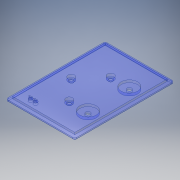
# Autodesk Inventor part: top
Saved by Autodesk Inventor 2017 SP1 (Build 210196100, 196)
## iProperties
Created: 2016-12-24
Part Number: top
Material: Generic
Document SubType Name: Modeling
Designer: wsh32
Density: 1 g/cm^3
Appearance: Clear - Blue
Author: wsh32
Autodesk Inventor part; units mm, degrees
ref_plane "YZ Plane" through (0, 0, 0) normal (1, 0, 0) x (0, 1, 0)
ref_plane "XZ Plane" through (0, 0, 0) normal (0, 1, 0) x (-1, 0, 0)
ref_plane "XY Plane" through (0, 0, 0) normal (0, 0, 1) x (1, 0, 0)
sketch "Sketch1" plane through (0, 0, 0) normal (0, 1, 0) x (-1, 0, 0)
  line L0 (0, 0) -> (-106.68, 0)
  line L1 (-106.68, 0) -> (-106.68, -153.67)
  line L2 (-106.68, -153.67) -> (0, -153.67)
  line L3 (0, -153.67) -> (0, 0)
  dimension "d0" = 153.67
  dimension "d1" = 106.68
  constraints: 8 end point, 2 parallel, 1 horizontal, 1 perpendicular
  measures "d0" distance of L2.end L0.start
  measures "d1" distance of L1.end L2.end
extrude "Extrusion1" add sketch "Sketch1" along normal blind 3.175
sketch "Sketch2" plane through (0, 3.175, 0) normal (0, 1, 0) x (1, 0, 0)
  line L0 (0, 0) -> (106.68, 0) projected
  line L1 (106.68, 0) -> (106.68, 153.67) projected
  line L2 (106.68, 153.67) -> (0, 153.67) projected
  line L3 (0, 153.67) -> (0, 0) projected
  line L4 (5.08, 5.08) -> (101.6, 5.08)
  line L5 (101.6, 5.08) -> (101.6, 148.59)
  line L6 (101.6, 148.59) -> (5.08, 148.59)
  line L7 (5.08, 148.59) -> (5.08, 5.08)
  dimension "d4" = 5.08
  constraints: 8 end point, 3 other
  measures "d4" distance between parallel lines of L3 L7
extrude "Extrusion2" add sketch "Sketch2" along normal blind 3.175 contours L7 L6 L5 L4
chamfer "Chamfer1" distance 1.27 angle 45 4 edges at (53.34, 0, 0) (0, 0, -76.835) (106.68, 0, -76.835) (53.34, 0, -153.67)
fillet "Fillet1" radius 3.175 4 edges at (0, 2.2225, -153.67) (0, 2.2225, 0) (106.68, 2.2225, 0) (106.68, 2.2225, -153.67)
sketch "Sketch6" plane through (0, 6.35, 0) normal (0, 1, 0) x (1, 0, 0)
  line L0 (5.08, 5.08) -> (101.6, 5.08) construction
  line L1 (101.6, 5.08) -> (101.6, 148.59) construction
  line L2 (101.6, 148.59) -> (5.08, 148.59) construction
  line L3 (5.08, 148.59) -> (5.08, 5.08) construction
  line L4 (53.34, 108.9244) -> (82.296, 108.9244) construction
  line L5 (82.296, 108.9244) -> (82.296, 44.7456) construction
  line L6 (82.296, 44.7456) -> (53.34, 44.7456) construction
  line L7 (53.34, 44.7456) -> (53.34, 108.9244) construction
  line L8 (53.34, 76.835) -> (82.296, 76.835) construction
  point P0 (0, 0)
  point P1 (24.384, 76.835)
  dimension "d39" = 39.6656
  dimension "d40" = 39.6656
  dimension "d41" = 64.1789
  dimension "d42" = 19.304
  dimension "d43" = 19.304
  dimension "d44" = 57.912
  dimension "d45" = 28.956
  dimension "d46" = 28.956
  constraints: 10 end point, 3 coincident, 2 midpoint, 2 parallel, 1 horizontal, 1 perpendicular, 1 point on line
  measures "d39" distance between parallel lines of L2 L4
  measures "d40" distance between parallel lines of L0 L6
  measures "d41" distance between parallel lines of L6 L4
  measures "d42" distance from line of L3 point (24.384, 76.835)
  measures "d43" distance between parallel lines of L1 L5
  measures "d44" distance from line of L5 point (24.384, 76.835)
  measures "d45" distance from line of point (24.384, 76.835) L7
  measures "d46" distance between parallel lines of L5 L7
hole "Hole3" at (53.34, 6.35, -108.9244) at (53.34, 6.35, -44.7456) at (24.384, 6.35, -76.835) direction (0, -1, 0) diameter 6.35 end through all counterbore diameter 10.16 counterbore depth 4.1275
sketch "Sketch7" plane through (0, 6.35, 0) normal (0, 1, 0) x (1, 0, 0)
  circle A0 centre (24.384, 76.835) radius 3.175 construction
  circle A1 centre (53.34, 108.9244) radius 3.175 construction
  circle A2 centre (53.34, 44.7456) radius 3.175 construction
  circle A3 centre (53.34, 108.9244) radius 3.175 construction
  line L0 (53.34, 108.9244) -> (82.296, 108.9244) construction
  line L1 (82.296, 108.9244) -> (82.296, 44.7456) construction
  line L2 (82.296, 44.7456) -> (53.34, 44.7456) construction
  line L3 (53.34, 44.7456) -> (53.34, 108.9244) construction
  point P0 (0, 0)
  dimension "d54" = 28.956
  dimension "d55" = 28.956
  constraints: 8 end point, 3 coincident, 2 parallel, 1 horizontal, 1 perpendicular
  measures "d54" distance from line of A0.centre L3
  measures "d55" distance between parallel lines of L1 L3
hole "Hole4" at (82.296, 6.35, -108.9244) at (82.296, 6.35, -44.7456) direction (0, -1, 0) diameter 6.985 end through all counterbore diameter 25.4 counterbore depth 3.81
sketch "Sketch8" plane through (0, 0, 0) normal (0, -1, 0) x (1, 0, 0)
  circle A0 centre (26.67, -19.05) radius 2.921
  circle A1 centre (19.05, -19.05) radius 2.921
  line L0 (26.67, -19.05) -> (19.05, -19.05) construction
  line L1 (0, -3.175) -> (0, -150.495) construction
  line L2 (103.505, 0) -> (3.175, 0) construction
  point P0 (0, 0)
  dimension "d63" = 5.842
  dimension "d64" = 7.62
  dimension "d65" = 19.05
  dimension "d66" = 19.05
  constraints: 2 centre point, 2 end point, 1 equal radius, 1 horizontal
  measures "d63" diameter of A1
  measures "d64" distance of L0.start L0.end
  measures "d65" distance from line of L1 L0.end
  measures "d66" distance between parallel lines of L2 L0
extrude "Extrusion4" cut sketch "Sketch8" against normal blind 3.175
sketch "Sketch9" plane through (26.67, 3.175, -19.05) normal (0, -1, 0) x (1, 0, 0)
  line L0 (0, 0) -> (-7.62, 0) construction
  circle A0 centre (0, 0) radius 2.921 construction
  circle A1 centre (-7.62, 0) radius 2.921 construction
  circle A2 centre (55.626, -89.8744) radius 3.4925 construction
  circle A3 centre (55.626, -25.6956) radius 3.4925 construction
  circle A4 centre (26.67, -25.6956) radius 3.175 construction
  circle A5 centre (26.67, -89.8744) radius 3.175 construction
  circle A6 centre (-2.286, -57.785) radius 3.175 construction
  line L1 (-25.4, 17.78) -> (78.74, 17.78) construction
  line L2 (-25.4, -133.35) -> (-25.4, 17.78) construction
  line L3 (78.74, -133.35) -> (-25.4, -133.35) construction
  line L4 (78.74, 17.78) -> (78.74, -133.35) construction
  point P0 (-26.67, 19.05)
  point P1 (1.5875, 0)
  point P2 (-1.5875, 0)
  point P3 (-6.0325, 0)
  point P4 (-9.2075, 0)
  dimension "d69" = 1.5875
  dimension "d70" = 1.5875
  dimension "d71" = 1.5875
  dimension "d72" = 1.5875
  dimension "d73" = 3.175
  constraints: 4 point on line, 2 coincident, 2 end point, 1 horizontal
  measures "d69" distance of L0.start point (1.587, 0)
  measures "d70" distance of L0.start point (-1.587, 0)
  measures "d71" distance of L0.end point (-6.032, 0)
  measures "d72" distance of L0.end point (-9.207, 0)
  measures "d73" distance of point (-1.587, 0) point (1.587, 0)
hole "Hole5" at (28.2575, 3.175, -19.05) at (25.0825, 3.175, -19.05) at (20.6375, 3.175, -19.05) at (17.4625, 3.175, -19.05) direction (0, 1, 0) diameter 2.032 end through all
equation "\"d40\" = d39"
equation "\"d41\" = 1.618 * d39"
equation "\"d43\" = d42"
equation "\"d44\" = 3 * d42"
equation "\"d46\" = d45"
equation "\"d55\" = d54"
equation "\"d70\" = d69"
equation "\"d71\" = d69"
equation "\"d72\" = d69"
body "Solid1"
